acrylic_inner_first_after_post_v8 (Autodesk Fusion 360 design; units mm, degrees)
Autodesk Fusion 360 part; units mm, degrees
note: some values were not read from the file. Chosen so that the rebuilt part matches the saved one: which bodies a step acts on.
sketch "Sketch1" plane through (0, 0, 0) normal (0, 1, 0) x (1, 0, 0)
  line L0 (193.9, 118.363) -> (193.9, 201.7255) construction
  line L1 (183.9, 190.7255) -> (183.9, 16)
  line L2 (23, 201.7255) -> (23, 118.363) construction
  line L3 (23, 12) -> (193.9, 12) construction
  circle A0 centre (23, 12) radius 1.5
  circle A1 centre (238.9, 12) radius 1.5
  line L4 (193.9, 95.3625) -> (23, 95.3625) construction
  line L5 (399.8, 190.7255) -> (399.8, 16)
  circle A2 centre (238.9, 95.3625) radius 1.5
  circle A3 centre (23, 201.7255) radius 1.5
  line L6 (33, 16) -> (33, 190.7255)
  line L7 (0, 212.7255) -> (0, 106.363) construction
  circle A4 centre (23, 118.363) radius 1.5
  circle A5 centre (193.9, 201.7255) radius 1.5
  circle A6 centre (23, 95.3625) radius 1.5
  line L8 (0, 106.3625) -> (0, 0) construction
  circle A7 centre (193.9, 95.3625) radius 1.5
  line L9 (23, 118.363) -> (193.9, 118.363) construction
  line L10 (193.9, 12) -> (193.9, 95.3625) construction
  circle A8 centre (193.9, 118.363) radius 1.5
  circle A9 centre (193.9, 12) radius 1.5
  line L11 (183.9, 16) -> (33, 16)
  line L12 (215.9, 0) -> (215.9, 106.3625) construction
  circle A10 centre (409.8, 118.363) radius 1.5
  line L13 (238.9, 118.363) -> (409.8, 118.363) construction
  line L14 (23, 95.3625) -> (23, 12) construction
  line L15 (215.9, 0) -> (431.8, 0) construction
  line L16 (431.8, 0) -> (431.8, 106.3625) construction
  line L17 (0, 106.363) -> (215.9, 106.363) construction
  circle A11 centre (409.8, 201.7255) radius 1.5
  line L18 (215.9, 106.3625) -> (0, 106.3625) construction
  line L19 (409.8, 201.7255) -> (238.9, 201.7255) construction
  line L20 (409.8, 12) -> (409.8, 95.3625) construction
  line L21 (215.9, 212.7255) -> (0, 212.7255) construction
  line L22 (0, 0) -> (215.9, 0) construction
  line L23 (215.9, 106.3625) -> (215.9, 0) construction
  circle A12 centre (409.8, 12) radius 1.5
  line L24 (215.9, 106.363) -> (431.8, 106.363) construction
  line L25 (409.8, 118.363) -> (409.8, 201.7255) construction
  line L26 (215.9, 106.363) -> (215.9, 212.7255) construction
  line L27 (238.9, 95.3625) -> (238.9, 12) construction
  circle A13 centre (409.8, 95.3625) radius 1.5
  line L28 (238.9, 12) -> (409.8, 12) construction
  line L29 (248.9, 16) -> (248.9, 190.7255)
  line L30 (248.9, 190.7255) -> (399.8, 190.7255)
  line L31 (431.8, 106.363) -> (431.8, 212.7255) construction
  line L32 (399.8, 16) -> (248.9, 16)
  line L33 (431.8, 212.7255) -> (215.9, 212.7255) construction
  line L34 (409.8, 95.3625) -> (238.9, 95.3625) construction
  line L35 (193.9, 201.7255) -> (23, 201.7255) construction
  line L36 (431.8, 106.3625) -> (215.9, 106.3625) construction
  line L37 (33, 190.7255) -> (183.9, 190.7255)
  circle A14 centre (238.9, 118.363) radius 1.5
  circle A15 centre (238.9, 201.7255) radius 1.5
  line L38 (238.9, 201.7255) -> (238.9, 118.363) construction
  line L39 (215.9, 212.7255) -> (215.9, 106.363) construction
  line L40 (432.8, 122.8753) -> (432.8, 213.7255)
  line L41 (432.8, 213.7255) -> (215.9, 213.7255)
  line L42 (215.9, 213.7255) -> (-1, 213.7255)
  line L43 (-1, 213.7255) -> (-1, 97.8373)
  line L44 (-1, 97.8373) -> (-1, -1)
  line L45 (-1, -1) -> (215.9, -1)
  line L46 (215.9, -1) -> (432.8, -1)
  line L47 (432.8, -1) -> (432.8, 122.8753)
  point P0 (215.9, 106.363)
  point P1 (0, 106.363)
  point P2 (215.9, 0)
  dimension "d3" = 215.9
  dimension "d4" = 106.363
  dimension "d5" = 106.3625
  dimension "d6" = 215.9
  dimension "d7" = 23
  dimension "d8" = 11
  dimension "d9" = 12
  dimension "d10" = 22
  dimension "d11" = 3
  dimension "d12" = 3
  dimension "d13" = 3
  dimension "d14" = 3
  dimension "d15" = 10
  dimension "d16" = 11
  dimension "d17" = 4
  dimension "d18" = 10
  dimension "d19" = 10
  dimension "d20" = 11
  dimension "d21" = 10
  dimension "d22" = 4
  dimension "d23" = 1
  dimension "d24" = 1
  constraint horizontal L22
  constraint vertical L12
  constraint horizontal L18
  constraint vertical L8
  constraint coincident L8.end L22.start
  constraint horizontal L3
  constraint vertical L10
  constraint horizontal L4
  constraint vertical L14
  constraint coincident L4.end A6.centre
  constraint coincident L3.start A0.centre
  constraint coincident L3.end L10.start
  constraint coincident L4.start A7.centre
  constraint horizontal L37
  constraint vertical L1
  constraint horizontal L11
  constraint vertical L6
  constraint horizontal L30
  constraint vertical L5
  constraint horizontal L32
  constraint vertical L29
  constraint coincident L43.end L44.start
  constraint coincident L40.start L47.end
  measures "d5" distance of L8.start L8.end
  measures "d6" distance of P2 L8.end
  measures "d7" distance of L8 L14
  measures "d8" distance of L4 L18
  measures "d9" distance of L3 L22
  measures "d10" distance of L10 L12
  measures "d11" diameter of A6
  measures "d12" diameter of A0
  measures "d13" diameter of A7
  measures "d14" diameter of A9
  measures "d15" distance of L2.end L6
  measures "d16" distance of L35 L37
  measures "d17" distance of L3 L11
  measures "d18" distance of L1 L10
  measures "d19" distance of L13.start L29
  measures "d20" distance of L19 L30
  measures "d21" distance of A11.centre L5
  measures "d22" distance of A1.centre L32
extrude "Extrude1" add sketch "Sketch1" along normal blind 5.4 makes body 1
sketch "Sketch2" plane through (0, 5.4, 0) normal (0, 1, 0) x (-1, 0, 0)
  circle A0 centre (-409.8, -12) radius 1.5
  circle A1 centre (-23, -95.3625) radius 1.5
  circle A2 centre (-409.8, -201.7255) radius 1.5
  circle A3 centre (-409.8, -95.3625) radius 1.5
  circle A4 centre (-238.9, -118.363) radius 1.5
  circle A5 centre (-238.9, -201.7255) radius 1.5
  circle A6 centre (-23, -12) radius 1.5
  circle A7 centre (-193.9, -201.7255) radius 1.5
  circle A8 centre (-193.9, -95.3625) radius 1.5
  line L0 (-399.8, -190.7255) -> (-399.8, -16)
  line L1 (-399.8, -16) -> (-248.9, -16)
  line L2 (-248.9, -16) -> (-248.9, -190.7255)
  line L3 (-248.9, -190.7255) -> (-399.8, -190.7255)
  circle A9 centre (-23, -201.7255) radius 1.5
  line L4 (-33, -16) -> (-33, -190.7255)
  line L5 (-33, -190.7255) -> (-183.9, -190.7255)
  line L6 (-183.9, -190.7255) -> (-183.9, -16)
  line L7 (-183.9, -16) -> (-33, -16)
  circle A10 centre (-23, -118.363) radius 1.5
  circle A11 centre (-238.9, -12) radius 1.5
  circle A12 centre (-238.9, -95.3625) radius 1.5
  circle A13 centre (-193.9, -118.363) radius 1.5
  circle A14 centre (-409.8, -118.363) radius 1.5
  circle A15 centre (-193.9, -12) radius 1.5
  line L8 (-432.8, 1) -> (-432.8, -122.8753)
  line L9 (-432.8, -122.8753) -> (-432.8, -213.7255)
  line L10 (-432.8, -213.7255) -> (1, -213.7255)
  line L11 (1, -213.7255) -> (1, -97.8373)
  line L12 (1, -97.8373) -> (1, 1)
  line L13 (1, 1) -> (-432.8, 1)
  line L14 (-399.8, -22) -> (-432.8, -22)
  line L15 (-432.8, -22) -> (-432.8, -82)
  line L16 (-432.8, -82) -> (-399.8, -82)
  line L17 (-399.8, -82) -> (-399.8, -22)
  dimension "d27" = 60
  dimension "d65" = 6
  dimension "d66" = 60
  constraint horizontal L14
  constraint vertical L15
  constraint horizontal L16
  constraint vertical L17
  constraint coincident L8.start L15
  measures "d27" distance of L14.start L16.end
  measures "d65" distance of L1 L14
  measures "d66" distance of L14 L16
extrude "Extrude2" cut sketch "Sketch2" against normal blind 20 contours L0 L8 L14 L15 L16 L17 bodies 1
sketch "Sketch3" plane through (0, 5.4, 0) normal (0, 1, 0) x (-1, 0, 0)
  circle A0 centre (-193.9, -12) radius 1.5
  circle A1 centre (-409.8, -118.363) radius 1.5
  circle A2 centre (-193.9, -118.363) radius 1.5
  circle A3 centre (-238.9, -95.3625) radius 1.5
  circle A4 centre (-238.9, -12) radius 1.5
  circle A5 centre (-23, -118.363) radius 1.5
  line L0 (-33, -16) -> (-33, -190.7255)
  line L1 (-33, -190.7255) -> (-183.9, -190.7255)
  line L2 (-183.9, -190.7255) -> (-183.9, -16)
  line L3 (-183.9, -16) -> (-33, -16)
  circle A6 centre (-23, -201.7255) radius 1.5
  line L4 (-432.8, -22) -> (-399.8, -22)
  line L5 (-248.9, -16) -> (-248.9, -190.7255)
  line L6 (-248.9, -190.7255) -> (-399.8, -190.7255)
  line L7 (-399.8, -22) -> (-399.8, -16)
  line L8 (-399.8, -82) -> (-432.8, -82)
  line L9 (-432.8, -82) -> (-432.8, -122.8753)
  line L10 (-432.8, -122.8753) -> (-432.8, -213.7255)
  line L11 (-432.8, -213.7255) -> (1, -213.7255)
  line L12 (1, -213.7255) -> (1, -97.8373)
  line L13 (1, -97.8373) -> (1, 1)
  line L14 (1, 1) -> (-432.8, 1)
  line L15 (-432.8, 1) -> (-432.8, -22)
  circle A7 centre (-193.9, -95.3625) radius 1.5
  circle A8 centre (-193.9, -201.7255) radius 1.5
  circle A9 centre (-23, -12) radius 1.5
  circle A10 centre (-238.9, -201.7255) radius 1.5
  circle A11 centre (-238.9, -118.363) radius 1.5
  circle A12 centre (-409.8, -95.3625) radius 1.5
  circle A13 centre (-409.8, -201.7255) radius 1.5
  circle A14 centre (-23, -95.3625) radius 1.5
  circle A15 centre (-409.8, -12) radius 1.5
  line L16 (1, -213.7255) -> (6.4, -213.7255)
  line L17 (6.4, -213.7255) -> (6.4, -193.7255)
  line L18 (6.4, -193.7255) -> (1, -193.7255)
  line L19 (1, -193.7255) -> (1, -213.7255)
  line L20 (1, 1) -> (6.4, 1)
  line L21 (6.4, 1) -> (6.4, -19)
  line L22 (6.4, -19) -> (1, -19)
  line L23 (1, -19) -> (1, 1)
  line L24 (1, 1) -> (-19, 1)
  line L25 (-19, 1) -> (-19, 6.4)
  line L26 (-19, 6.4) -> (1, 6.4)
  line L27 (1, 6.4) -> (1, 1)
  line L28 (1, -213.7255) -> (-19, -213.7255)
  line L29 (-19, -213.7255) -> (-19, -219.1255)
  line L30 (-19, -219.1255) -> (1, -219.1255)
  line L31 (1, -219.1255) -> (1, -213.7255)
  line L32 (-432.8, -213.7255) -> (-412.8, -213.7255)
  line L33 (-412.8, -213.7255) -> (-412.8, -219.1255)
  line L34 (-412.8, -219.1255) -> (-432.8, -219.1255)
  line L35 (-432.8, -219.1255) -> (-432.8, -213.7255)
  line L36 (-432.8, -213.7255) -> (-438.2, -213.7255)
  line L37 (-438.2, -213.7255) -> (-438.2, -193.7255)
  line L38 (-438.2, -193.7255) -> (-432.8, -193.7255)
  line L39 (-432.8, -193.7255) -> (-432.8, -213.7255)
  line L40 (-432.8, 1) -> (-438.2, 1)
  line L41 (-438.2, 1) -> (-438.2, -19)
  line L42 (-438.2, -19) -> (-432.8, -19)
  line L43 (-432.8, -19) -> (-432.8, 1)
  line L44 (-432.8, 1) -> (-412.8, 1)
  line L45 (-412.8, 1) -> (-412.8, 6.4)
  line L46 (-412.8, 6.4) -> (-432.8, 6.4)
  line L47 (-432.8, 6.4) -> (-432.8, 1)
  line L48 (-205.9, 1) -> (-225.9, 1)
  line L49 (-225.9, 1) -> (-225.9, 6.4)
  line L50 (-225.9, 6.4) -> (-205.9, 6.4)
  line L51 (-205.9, 6.4) -> (-205.9, 1)
  line L52 (-205.9, -213.7255) -> (-225.9, -213.7255)
  line L53 (-225.9, -213.7255) -> (-225.9, -219.1255)
  line L54 (-225.9, -219.1255) -> (-205.9, -219.1255)
  line L55 (-205.9, -219.1255) -> (-205.9, -213.7255)
  line L56 (-399.8, -16) -> (-248.9, -16)
  line L57 (-399.8, -190.7255) -> (-399.8, -82)
  dimension "d30" = 5.4
  dimension "d31" = 20
  dimension "d32" = 5.4
  dimension "d33" = 20
  dimension "d34" = 20
  dimension "d35" = 5.4
  dimension "d36" = 5.4
  dimension "d37" = 20
  dimension "d38" = 20
  dimension "d39" = 5.4
  dimension "d40" = 5.4
  dimension "d41" = 20
  dimension "d42" = 5.4
  dimension "d43" = 20
  dimension "d44" = 20
  dimension "d45" = 5.4
  dimension "d46" = 20
  dimension "d47" = 5.4
  dimension "d48" = 20
  dimension "d49" = 5.4
  dimension "d50" = 206.9
  dimension "d51" = 206.9
  dimension "d63" = 433.8
  constraint horizontal L16
  constraint vertical L17
  constraint horizontal L18
  constraint vertical L19
  constraint coincident L11.end L12.start
  constraint horizontal L20
  constraint vertical L21
  constraint horizontal L22
  constraint vertical L23
  constraint coincident L13.end L14.start
  constraint horizontal L24
  constraint vertical L25
  constraint horizontal L26
  constraint vertical L27
  constraint horizontal L28
  constraint vertical L29
  constraint horizontal L30
  constraint vertical L31
  constraint horizontal L32
  constraint vertical L33
  constraint horizontal L34
  constraint vertical L35
  constraint coincident L10.end L11.start
  constraint horizontal L36
  constraint vertical L37
  constraint horizontal L38
  constraint vertical L39
  constraint horizontal L40
  constraint vertical L41
  constraint horizontal L42
  constraint vertical L43
  constraint coincident L14.end L15.start
  constraint horizontal L44
  constraint vertical L45
  constraint horizontal L46
  constraint vertical L47
  constraint horizontal L48
  constraint vertical L49
  constraint horizontal L50
  constraint vertical L51
  constraint coincident L14 L48.start
  constraint horizontal L52
  constraint vertical L53
  constraint horizontal L54
  constraint vertical L55
  constraint coincident L11 L52.start
  measures "d30" distance of L13.end L20.end
  measures "d31" distance of L20.end L21.end
  measures "d32" distance of L11.end L16.end
  measures "d33" distance of L16.end L17.end
  measures "d34" distance of L13.end L24.end
  measures "d35" distance of L13.end L26.end
  measures "d36" distance of L11.end L30.end
  measures "d37" distance of L29.end L30.end
  measures "d38" distance of L10.end L32.end
  measures "d39" distance of L10.end L34.end
  measures "d40" distance of L10.end L36.end
  measures "d41" distance of L10.end L38.end
  measures "d42" distance of L14.end L40.end
  measures "d43" distance of L14.end L42.end
  measures "d44" distance of L14.end L44.end
  measures "d45" distance of L14.end L46.end
  measures "d46" distance of L48.start L48.end
  measures "d47" distance of L48.start L50.end
  measures "d48" distance of L52.start L52.end
  measures "d49" distance of L52.start L54.end
  measures "d50" distance of L12 L55
  measures "d51" distance of L13 L51
  measures "d63" distance of L10 L12
extrude "Extrude3" add sketch "Sketch3" against normal blind 5.4 contours L15 L40 L41 L42 L43 | L14 L44 L45 L46 L47 | L14 L48 L49 L50 L51 | L14 L24 L25 L26 L27 | L13 L20 L21 L22 L23 | L10 L36 L37 L38 L39 | L11 L32 L33 L34 L35 | L12 L16 L17 L18 L19 | L11 L28 L29 L30 L31 | L11 L52 L53 L54 L55 bodies 1
sketch "Sketch4" plane through (0, 5.4, 0) normal (0, 1, 0) x (-1, 0, 0)
  circle A0 centre (-193.9, -12) radius 1.5
  circle A1 centre (-409.8, -118.363) radius 1.5
  circle A2 centre (-193.9, -118.363) radius 1.5
  circle A3 centre (-238.9, -95.3625) radius 1.5
  circle A4 centre (-238.9, -12) radius 1.5
  circle A5 centre (-23, -118.363) radius 1.5
  line L0 (-33, -16) -> (-33, -190.7255)
  line L1 (-33, -190.7255) -> (-183.9, -190.7255)
  line L2 (-183.9, -190.7255) -> (-183.9, -16)
  line L3 (-183.9, -16) -> (-33, -16)
  circle A6 centre (-23, -201.7255) radius 1.5
  line L4 (-432.8, -22) -> (-399.8, -22)
  line L5 (-248.9, -16) -> (-248.9, -190.7255)
  line L6 (-248.9, -190.7255) -> (-399.8, -190.7255)
  line L7 (-399.8, -22) -> (-399.8, -16)
  line L8 (-399.8, -82) -> (-432.8, -82)
  line L9 (-432.8, -82) -> (-432.8, -122.8753)
  line L10 (-432.8, -122.8753) -> (-432.8, -193.7255)
  line L11 (-432.8, -193.7255) -> (-438.2, -193.7255)
  line L12 (-438.2, -193.7255) -> (-438.2, -213.7255)
  line L13 (-438.2, -213.7255) -> (-432.8, -213.7255)
  line L14 (-432.8, -213.7255) -> (-432.8, -219.1255)
  line L15 (-432.8, -219.1255) -> (-412.8, -219.1255)
  line L16 (-412.8, -219.1255) -> (-412.8, -213.7255)
  line L17 (-412.8, -213.7255) -> (-225.9, -213.7255)
  line L18 (-225.9, -213.7255) -> (-225.9, -219.1255)
  line L19 (-225.9, -219.1255) -> (-205.9, -219.1255)
  line L20 (-205.9, -219.1255) -> (-205.9, -213.7255)
  line L21 (-205.9, -213.7255) -> (-19, -213.7255)
  line L22 (-19, -213.7255) -> (-19, -219.1255)
  line L23 (-19, -219.1255) -> (1, -219.1255)
  line L24 (1, -219.1255) -> (1, -213.7255)
  line L25 (1, -213.7255) -> (6.4, -213.7255)
  line L26 (6.4, -213.7255) -> (6.4, -193.7255)
  line L27 (6.4, -193.7255) -> (1, -193.7255)
  line L28 (1, -193.7255) -> (1, -97.8373)
  line L29 (1, -97.8373) -> (1, -19)
  line L30 (1, -19) -> (6.4, -19)
  line L31 (6.4, -19) -> (6.4, 1)
  line L32 (6.4, 1) -> (1, 1)
  line L33 (1, 1) -> (1, 6.4)
  line L34 (1, 6.4) -> (-19, 6.4)
  line L35 (-19, 6.4) -> (-19, 1)
  line L36 (-19, 1) -> (-205.9, 1)
  line L37 (-205.9, 1) -> (-205.9, 6.4)
  line L38 (-205.9, 6.4) -> (-225.9, 6.4)
  line L39 (-225.9, 6.4) -> (-225.9, 1)
  line L40 (-225.9, 1) -> (-412.8, 1)
  line L41 (-412.8, 1) -> (-412.8, 6.4)
  line L42 (-412.8, 6.4) -> (-432.8, 6.4)
  line L43 (-432.8, 6.4) -> (-432.8, 1)
  line L44 (-432.8, 1) -> (-438.2, 1)
  line L45 (-438.2, 1) -> (-438.2, -19)
  line L46 (-438.2, -19) -> (-432.8, -19)
  line L47 (-432.8, -19) -> (-432.8, -22)
  circle A7 centre (-193.9, -95.3625) radius 1.5
  circle A8 centre (-193.9, -201.7255) radius 1.5
  circle A9 centre (-23, -12) radius 1.5
  circle A10 centre (-238.9, -201.7255) radius 1.5
  circle A11 centre (-238.9, -118.363) radius 1.5
  circle A12 centre (-409.8, -95.3625) radius 1.5
  circle A13 centre (-409.8, -201.7255) radius 1.5
  circle A14 centre (-23, -95.3625) radius 1.5
  circle A15 centre (-409.8, -12) radius 1.5
  line L48 (1, -116.3627) -> (6.4, -116.3627)
  line L49 (6.4, -116.3627) -> (6.4, -96.3627)
  line L50 (6.4, -96.3627) -> (1, -96.3627)
  line L51 (1, -96.3627) -> (1, -116.3627)
  line L52 (-215.9, 6.4) -> (-215.9, -219.1255) construction
  line L53 (-432.8, -116.3627) -> (-438.2, -116.3627)
  line L54 (-438.2, -116.3627) -> (-438.2, -96.3627)
  line L55 (-438.2, -96.3627) -> (-432.8, -96.3627)
  line L56 (-432.8, -96.3627) -> (-432.8, -116.3627)
  line L57 (-399.8, -16) -> (-248.9, -16)
  line L58 (-399.8, -190.7255) -> (-399.8, -82)
  dimension "d54" = 20
  dimension "d55" = 5.4
  dimension "d56" = 174.7255
  dimension "d57" = 77.3628
  dimension "d58" = 5.4
  dimension "d59" = 20
  dimension "d64" = 77.3628
  dimension "d80" = 20
  dimension "d81" = 5.4
  constraint horizontal L48
  constraint vertical L49
  constraint horizontal L50
  constraint vertical L51
  constraint coincident L28 L48.start
  constraint midpoint L38 L52.start
  constraint midpoint L19 L52.end
  constraint horizontal L53
  constraint vertical L54
  constraint horizontal L55
  constraint vertical L56
  constraint coincident L9 L53.start
  measures "d54" distance of L48.end L49.end
  measures "d55" distance of L49.end L50.end
  measures "d56" distance of L26.end L30.end
  measures "d57" distance of L30.end L49.end
  measures "d58" distance of L53.start L53.end
  measures "d59" distance of L53.start L55.end
  measures "d64" distance of L45.end L54.end
  measures "d80" distance of L25.end L26.end
  measures "d81" distance of L24.end L25.end
extrude "Extrude4" add sketch "Sketch4" against normal blind 5.4 contours L9 L53 L54 L55 L56 | L28 L29 L48 L49 L50 L51 bodies 1
sketch "Sketch5" plane through (0, 5.4, 0) normal (0, 1, 0) x (-1, 0, 0)
  circle A0 centre (-409.8, -95.3625) radius 1.5
  line L0 (-33, -16) -> (-33, -190.7255)
  line L1 (-33, -190.7255) -> (-183.9, -190.7255)
  line L2 (-183.9, -190.7255) -> (-183.9, -16)
  line L3 (-183.9, -16) -> (-33, -16)
  circle A1 centre (-238.9, -118.363) radius 1.5
  circle A2 centre (-409.8, -118.363) radius 1.5
  circle A3 centre (-409.8, -12) radius 1.5
  circle A4 centre (-238.9, -12) radius 1.5
  circle A5 centre (-238.9, -95.3625) radius 1.5
  circle A6 centre (-409.8, -201.7255) radius 1.5
  circle A7 centre (-193.9, -12) radius 1.5
  circle A8 centre (-193.9, -118.363) radius 1.5
  circle A9 centre (-193.9, -201.7255) radius 1.5
  circle A10 centre (-193.9, -95.3625) radius 1.5
  circle A11 centre (-23, -95.3625) radius 1.5
  circle A12 centre (-23, -12) radius 1.5
  circle A13 centre (-23, -118.363) radius 1.5
  circle A14 centre (-23, -201.7255) radius 1.5
  circle A15 centre (-238.9, -201.7255) radius 1.5
  line L4 (-432.8, -22) -> (-399.8, -22)
  line L5 (-399.8, -22) -> (-399.8, -16)
  line L6 (-399.8, -16) -> (-248.9, -16)
  line L7 (-248.9, -16) -> (-248.9, -190.7255)
  line L8 (-248.9, -190.7255) -> (-399.8, -190.7255)
  line L9 (-399.8, -190.7255) -> (-399.8, -82)
  line L10 (-399.8, -82) -> (-432.8, -82)
  line L11 (-432.8, -82) -> (-432.8, -96.3627)
  line L12 (-432.8, -96.3627) -> (-438.2, -96.3627)
  line L13 (-438.2, -96.3627) -> (-438.2, -116.3627)
  line L14 (-438.2, -116.3627) -> (-432.8, -116.3627)
  line L15 (-432.8, -116.3627) -> (-432.8, -122.8753)
  line L16 (-432.8, -122.8753) -> (-432.8, -193.7255)
  line L17 (-432.8, -193.7255) -> (-438.2, -193.7255)
  line L18 (-438.2, -193.7255) -> (-438.2, -213.7255)
  line L19 (-438.2, -213.7255) -> (-432.8, -213.7255)
  line L20 (-432.8, -213.7255) -> (-432.8, -219.1255)
  line L21 (-432.8, -219.1255) -> (-412.8, -219.1255)
  line L22 (-412.8, -219.1255) -> (-412.8, -213.7255)
  line L23 (-412.8, -213.7255) -> (-225.9, -213.7255)
  line L24 (-225.9, -213.7255) -> (-225.9, -219.1255)
  line L25 (-225.9, -219.1255) -> (-205.9, -219.1255)
  line L26 (-205.9, -219.1255) -> (-205.9, -213.7255)
  line L27 (-205.9, -213.7255) -> (-19, -213.7255)
  line L28 (-19, -213.7255) -> (-19, -219.1255)
  line L29 (-19, -219.1255) -> (1, -219.1255)
  line L30 (1, -219.1255) -> (1, -213.7255)
  line L31 (1, -213.7255) -> (6.4, -213.7255)
  line L32 (6.4, -213.7255) -> (6.4, -193.7255)
  line L33 (6.4, -193.7255) -> (1, -193.7255)
  line L34 (1, -193.7255) -> (1, -116.3627)
  line L35 (1, -116.3627) -> (6.4, -116.3627)
  line L36 (6.4, -116.3627) -> (6.4, -96.3627)
  line L37 (6.4, -96.3627) -> (1, -96.3627)
  line L38 (1, -96.3627) -> (1, -19)
  line L39 (1, -19) -> (6.4, -19)
  line L40 (6.4, -19) -> (6.4, 1)
  line L41 (6.4, 1) -> (1, 1)
  line L42 (1, 1) -> (1, 6.4)
  line L43 (1, 6.4) -> (-19, 6.4)
  line L44 (-19, 6.4) -> (-19, 1)
  line L45 (-19, 1) -> (-205.9, 1)
  line L46 (-205.9, 1) -> (-205.9, 6.4)
  line L47 (-205.9, 6.4) -> (-225.9, 6.4)
  line L48 (-225.9, 6.4) -> (-225.9, 1)
  line L49 (-225.9, 1) -> (-412.8, 1)
  line L50 (-412.8, 1) -> (-412.8, 6.4)
  line L51 (-412.8, 6.4) -> (-432.8, 6.4)
  line L52 (-432.8, 6.4) -> (-432.8, 1)
  line L53 (-432.8, 1) -> (-438.2, 1)
  line L54 (-438.2, 1) -> (-438.2, -19)
  line L55 (-438.2, -19) -> (-432.8, -19)
  line L56 (-432.8, -19) -> (-432.8, -22)
  line L57 (-183.9, -160.7255) -> (-248.9, -160.7255)
  line L58 (-248.9, -160.7255) -> (-248.9, -125.7255)
  line L59 (-248.9, -125.7255) -> (-183.9, -125.7255)
  line L60 (-183.9, -125.7255) -> (-183.9, -160.7255)
  line L61 (-183.9, -70.7255) -> (-248.9, -70.7255)
  line L62 (-248.9, -70.7255) -> (-248.9, -35.7255)
  line L63 (-248.9, -35.7255) -> (-183.9, -35.7255)
  line L64 (-183.9, -35.7255) -> (-183.9, -70.7255)
  dimension "d67" = 30
  dimension "d68" = 65
  dimension "d69" = 120
  dimension "d70" = 35
  constraint horizontal L57
  constraint vertical L58
  constraint horizontal L59
  constraint vertical L60
  constraint coincident L7 L58.end
  constraint coincident L2 L57.start
  constraint horizontal L61
  constraint vertical L62
  constraint horizontal L63
  constraint vertical L64
  constraint coincident L7 L62.end
  constraint coincident L2 L61.start
  measures "d67" distance of L1 L57
  measures "d68" distance of L1 L59
  measures "d69" distance of L1 L61
  measures "d70" distance of L61 L63
extrude "Extrude5" cut sketch "Sketch5" against normal blind 40 contours L2 L7 L61 L62 L63 L64 | L2 L7 L57 L58 L59 L60 bodies 1 makes body 2 at (223.4955, 0, -174.0983)
sketch "Sketch6" plane through (0, 5.4, 0) normal (0, 1, 0) x (-1, 0, 0)
  line L0 (-248.9, -125.7255) -> (-183.9, -125.7255)
  line L1 (-183.9, -125.7255) -> (-183.9, -70.7255)
  line L2 (-183.9, -70.7255) -> (-248.9, -70.7255)
  line L3 (-248.9, -70.7255) -> (-248.9, -125.7255)
  circle A0 centre (-238.9, -118.363) radius 1.5
  circle A1 centre (-238.9, -95.3625) radius 1.5
  circle A2 centre (-193.9, -118.363) radius 1.5
  circle A3 centre (-193.9, -95.3625) radius 1.5
  line L4 (-183.9, -123.2713) -> (-33, -123.2713)
  line L5 (-33, -123.2713) -> (-33, -85.5458)
  line L6 (-33, -85.5458) -> (-183.9, -85.5458)
  line L7 (-183.9, -85.5458) -> (-183.9, -123.2713)
  line L8 (-248.9, -123.2713) -> (-399.8, -123.2713)
  line L9 (-399.8, -123.2713) -> (-399.8, -85.5458)
  line L10 (-399.8, -85.5458) -> (-248.9, -85.5458)
  line L11 (-248.9, -85.5458) -> (-248.9, -125.7255)
  line L12 (-399.8, -190.7255) -> (-399.8, -82) construction
  line L13 (-33, -16) -> (-33, -190.7255) construction
  dimension "d74" = 9.8167
  dimension "d75" = 9.8167
  dimension "d78" = 7.3625
  dimension "d79" = 4.9083
  constraint horizontal L4
  constraint vertical L5
  constraint horizontal L6
  constraint vertical L7
  constraint horizontal L8
  constraint vertical L9
  constraint horizontal L10
  constraint vertical L11
  constraint coincident L8.end L12
  constraint coincident L4.end L13
  constraint collinear L4 L8
  constraint coincident L11 L8.start
  constraint coincident L4.start L7.end
  constraint coincident L0.start L3.end
  constraint coincident L0.start L11
  constraint coincident L0.end L7
  measures "d74" distance of A3.centre L6
  measures "d75" distance of A1.centre L10
  measures "d78" distance of L0 A2.centre
  measures "d79" distance of A2.centre L4
extrude "Extrude6" add sketch "Sketch6" against normal blind 5.4 contours L3 L8 L9 L10 L11 | L1 L4 L5 L6 L7 bodies 1 2
sketch "export" plane through (0, 5.4, 0) normal (0, 1, 0) x (-1, 0, 0)
  line L0 (-399.8, -85.5458) -> (-399.8, -82)
  line L1 (-399.8, -82) -> (-432.8, -82)
  line L2 (-432.8, -82) -> (-432.8, -96.3627)
  line L3 (-432.8, -96.3627) -> (-438.2, -96.3627)
  line L4 (-438.2, -96.3627) -> (-438.2, -116.3627)
  line L5 (-438.2, -116.3627) -> (-432.8, -116.3627)
  line L6 (-432.8, -116.3627) -> (-432.8, -122.8753)
  line L7 (-432.8, -122.8753) -> (-432.8, -193.7255)
  line L8 (-432.8, -193.7255) -> (-438.2, -193.7255)
  line L9 (-438.2, -193.7255) -> (-438.2, -213.7255)
  line L10 (-438.2, -213.7255) -> (-432.8, -213.7255)
  line L11 (-432.8, -213.7255) -> (-432.8, -219.1255)
  line L12 (-432.8, -219.1255) -> (-412.8, -219.1255)
  line L13 (-412.8, -219.1255) -> (-412.8, -213.7255)
  line L14 (-412.8, -213.7255) -> (-225.9, -213.7255)
  line L15 (-225.9, -213.7255) -> (-225.9, -219.1255)
  line L16 (-225.9, -219.1255) -> (-205.9, -219.1255)
  line L17 (-205.9, -219.1255) -> (-205.9, -213.7255)
  line L18 (-205.9, -213.7255) -> (-19, -213.7255)
  line L19 (-19, -213.7255) -> (-19, -219.1255)
  line L20 (-19, -219.1255) -> (1, -219.1255)
  line L21 (1, -219.1255) -> (1, -213.7255)
  line L22 (1, -213.7255) -> (6.4, -213.7255)
  line L23 (6.4, -213.7255) -> (6.4, -193.7255)
  line L24 (6.4, -193.7255) -> (1, -193.7255)
  line L25 (1, -193.7255) -> (1, -116.3627)
  line L26 (1, -116.3627) -> (6.4, -116.3627)
  line L27 (6.4, -116.3627) -> (6.4, -96.3627)
  line L28 (6.4, -96.3627) -> (1, -96.3627)
  line L29 (1, -96.3627) -> (1, -19)
  line L30 (1, -19) -> (6.4, -19)
  line L31 (6.4, -19) -> (6.4, 1)
  line L32 (6.4, 1) -> (1, 1)
  line L33 (1, 1) -> (1, 6.4)
  line L34 (1, 6.4) -> (-19, 6.4)
  line L35 (-19, 6.4) -> (-19, 1)
  line L36 (-19, 1) -> (-205.9, 1)
  line L37 (-205.9, 1) -> (-205.9, 6.4)
  line L38 (-205.9, 6.4) -> (-225.9, 6.4)
  line L39 (-225.9, 6.4) -> (-225.9, 1)
  line L40 (-225.9, 1) -> (-412.8, 1)
  line L41 (-412.8, 1) -> (-412.8, 6.4)
  line L42 (-412.8, 6.4) -> (-432.8, 6.4)
  line L43 (-432.8, 6.4) -> (-432.8, 1)
  line L44 (-432.8, 1) -> (-438.2, 1)
  line L45 (-438.2, 1) -> (-438.2, -19)
  line L46 (-438.2, -19) -> (-432.8, -19)
  line L47 (-432.8, -19) -> (-432.8, -22)
  line L48 (-432.8, -22) -> (-399.8, -22)
  line L49 (-399.8, -22) -> (-399.8, -16)
  line L50 (-399.8, -16) -> (-248.9, -16)
  line L51 (-248.9, -16) -> (-248.9, -35.7255)
  line L52 (-248.9, -35.7255) -> (-183.9, -35.7255)
  line L53 (-183.9, -35.7255) -> (-183.9, -16)
  line L54 (-183.9, -16) -> (-33, -16)
  line L55 (-33, -16) -> (-33, -85.5458)
  line L56 (-33, -85.5458) -> (-183.9, -85.5458)
  line L57 (-183.9, -85.5458) -> (-183.9, -70.7255)
  line L58 (-183.9, -70.7255) -> (-248.9, -70.7255)
  line L59 (-248.9, -70.7255) -> (-248.9, -85.5458)
  line L60 (-248.9, -85.5458) -> (-399.8, -85.5458)
  circle A0 centre (-409.8, -95.3625) radius 1.5
  circle A1 centre (-409.8, -118.363) radius 1.5
  circle A2 centre (-409.8, -12) radius 1.5
  circle A3 centre (-238.9, -12) radius 1.5
  circle A4 centre (-409.8, -201.7255) radius 1.5
  circle A5 centre (-193.9, -12) radius 1.5
  circle A6 centre (-193.9, -201.7255) radius 1.5
  circle A7 centre (-23, -95.3625) radius 1.5
  circle A8 centre (-23, -12) radius 1.5
  circle A9 centre (-23, -118.363) radius 1.5
  circle A10 centre (-23, -201.7255) radius 1.5
  circle A11 centre (-238.9, -201.7255) radius 1.5
  line L61 (-399.8, -123.2713) -> (-248.9, -123.2713)
  line L62 (-248.9, -123.2713) -> (-248.9, -125.7255)
  line L63 (-248.9, -125.7255) -> (-183.9, -125.7255)
  line L64 (-183.9, -125.7255) -> (-183.9, -123.2713)
  line L65 (-183.9, -123.2713) -> (-33, -123.2713)
  line L66 (-33, -123.2713) -> (-33, -190.7255)
  line L67 (-33, -190.7255) -> (-183.9, -190.7255)
  line L68 (-183.9, -190.7255) -> (-183.9, -160.7255)
  line L69 (-183.9, -160.7255) -> (-248.9, -160.7255)
  line L70 (-248.9, -160.7255) -> (-248.9, -190.7255)
  line L71 (-248.9, -190.7255) -> (-399.8, -190.7255)
  line L72 (-399.8, -190.7255) -> (-399.8, -123.2713)
  circle A12 centre (-238.9, -118.363) radius 1.5
  circle A13 centre (-238.9, -95.3625) radius 1.5
  circle A14 centre (-193.9, -118.363) radius 1.5
  circle A15 centre (-193.9, -95.3625) radius 1.5
equation "d11 = d12"
equation "d13 = d12"
equation "d14 = d12"
equation "d17 = 11.00 mm - 7 mm"
equation "d22 = d17"
equation "d30 = d36"
equation "d31 = d33"
equation "d32 = d36"
equation "d34 = d33"
equation "d35 = d36"
equation "d37 = d33"
equation "d38 = d33"
equation "d39 = d36"
equation "d40 = d36"
equation "d41 = d33"
equation "d42 = d36"
equation "d43 = d33"
equation "d44 = d33"
equation "d45 = d32"
equation "d46 = d33"
equation "d47 = d36"
equation "d48 = d33"
equation "d49 = d36"
equation "d50 = ( d63 - d48 ) / 2"
equation "d51 = d50"
equation "d54 = d80"
equation "d55 = d81"
equation "d57 = ( d56 - d54 ) / 2"
equation "d58 = d55"
equation "d59 = d54"
equation "d64 = d57"
equation "d66 = d27"
equation "d70 = d68 - d67"
equation "d74 = 2 * d79"
equation "d75 = d74"
equation "d79 = 2 * d78 / 3"
